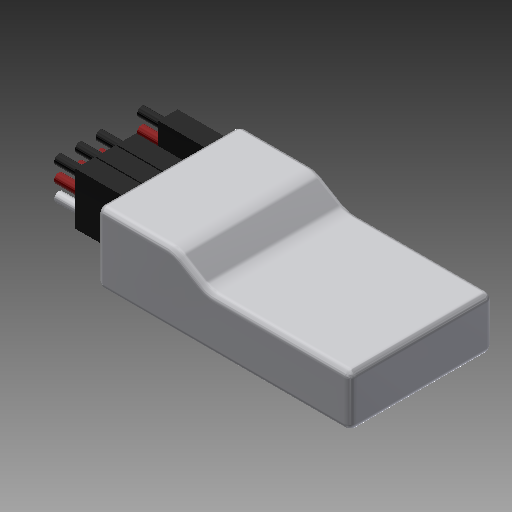
# Autodesk Inventor part: 受信機
Saved by Autodesk Inventor 2020 (Build 240168000, 168)
## iProperties
Created: 2013-08-05
Part Number: 受信機
Material: 一般
Document SubType Name: Modeling
Designer: Kentaro2
Mass: 5 g
Surface Area: 27.3811 cm^2
Volume: 7.76151 cm^3
Density: 0.644204 g/cm^3
Appearance: 既定
Author: Kentaro2
Autodesk Inventor part; units mm, degrees
ref_plane "YZ Plane" through (0, 0, 0) normal (1, 0, 0) x (0, 1, 0)
ref_plane "XZ Plane" through (0, 0, 0) normal (0, 1, 0) x (-1, 0, 0)
ref_plane "XY Plane" through (0, 0, 0) normal (0, 0, 1) x (1, 0, 0)
sketch "スケッチ1" plane through (0, 0, 0) normal (0, 0, 1) x (1, 0, 0)
  line L0 (-19.5, 11) -> (-19.5, 0)
  line L1 (-19.5, 0) -> (19.5, 0)
  line L2 (19.5, 0) -> (19.5, 8)
  line L3 (19.5, 8) -> (-2.5, 8)
  line L4 (-2.5, 8) -> (-7.5, 11)
  line L5 (-7.5, 11) -> (-19.5, 11)
  point P0 (0, 0)
  point P1 (0, 0)
  dimension "d0" = 8
  dimension "d1" = 11
  dimension "d2" = 39
  dimension "d3" = 12
  dimension "d4" = 22
  constraints: 12 end point, 3 parallel, 1 coincident, 1 horizontal, 1 midpoint, 1 perpendicular
  measures "d0" distance between parallel lines of L1 L3
  measures "d1" distance between parallel lines of L1 L5
  measures "d2" distance between parallel lines of L2 L0
  measures "d3" distance of L4.end L0.start
  measures "d4" distance of L2.end L3.end
extrude "押し出し1" add sketch "スケッチ1" along normal blind 22
fillet "フィレット1" radius 1 16 edges at (0, 0, 22) (8.5, 8, 22) (19.5, 4, 22) (-19.5, 0, 11) (0, 0, 0) (19.5, 0, 11) (19.5, 4, 0) (19.5, 8, 11) (-5, 9.5, 22) (8.5, 8, 0) (-5, 9.5, 0) (-13.5, 11, 22) (-19.5, 5.5, 22) (-13.5, 11, 0) (-19.5, 5.5, 0) (-19.5, 11, 11)
fillet "フィレット1" radius 4 2 edges at (-7.5, 11, 11) (-2.5, 8, 11)
sketch "スケッチ2" plane through (-19.5, 1, 1) normal (-1, 0, 0) x (0, 0, 1)
  line L0 (0, 0) -> (0, 9) projected
  line L1 (20, 0) -> (0, 0) projected
  line L2 (20, 9) -> (20, 0) projected
  line L3 (0.5347, 8.5347) -> (0.5347, 0.5347)
  line L4 (0.5347, 0.5347) -> (19.4653, 0.5347)
  line L5 (19.4653, 0.5347) -> (19.4653, 8.5)
  line L6 (0.5347, 8.5347) -> (3.5347, 8.5347)
  line L7 (3.5347, 8.5347) -> (3.5347, 0.5347)
  line L8 (3.5347, 0.5347) -> (0.5347, 0.5347)
  line L9 (0.5347, 0.5347) -> (0.5347, 8.5347)
  line L10 (3.7208, 8.5347) -> (6.7208, 8.5347)
  line L11 (6.7208, 8.5347) -> (6.7208, 0.5347)
  line L12 (6.7208, 0.5347) -> (3.7208, 0.5347)
  line L13 (3.7208, 0.5347) -> (3.7208, 8.5347)
  line L14 (6.9069, 8.5347) -> (9.9069, 8.5347)
  line L15 (9.9069, 8.5347) -> (9.9069, 0.5347)
  line L16 (9.9069, 0.5347) -> (6.9069, 0.5347)
  line L17 (6.9069, 0.5347) -> (6.9069, 8.5347)
  line L18 (10.0931, 8.5347) -> (13.0931, 8.5347)
  line L19 (13.0931, 8.5347) -> (13.0931, 0.5347)
  line L20 (13.0931, 0.5347) -> (10.0931, 0.5347)
  line L21 (10.0931, 0.5347) -> (10.0931, 8.5347)
  line L22 (13.2792, 8.5347) -> (16.2792, 8.5347)
  line L23 (16.2792, 8.5347) -> (16.2792, 0.5347)
  line L24 (16.2792, 0.5347) -> (13.2792, 0.5347)
  line L25 (13.2792, 0.5347) -> (13.2792, 8.5347)
  line L26 (16.4653, 8.5347) -> (19.4653, 8.5347)
  line L27 (19.4653, 8.5347) -> (19.4653, 0.5347)
  line L28 (19.4653, 0.5347) -> (16.4653, 0.5347)
  line L29 (16.4653, 0.5347) -> (16.4653, 8.5347)
  line L30 (3.5347, 8.5347) -> (3.7208, 8.5347)
  line L31 (6.7208, 8.5347) -> (6.9069, 8.5347)
  line L32 (9.9069, 8.5347) -> (10.0931, 8.5347)
  line L33 (13.0931, 8.5347) -> (13.2792, 8.5347)
  line L34 (16.2792, 8.5347) -> (16.4653, 8.5347)
  point P0 (-1, -1)
  dimension "d9" = 8
  dimension "d11" = 0.5347
  dimension "d12" = 3
  constraints: 64 end point, 16 equal length, 9 collinear, 7 perpendicular, 6 horizontal, 5 point on line, 2 other
  measures "d9" distance of L3.start L3.end
  measures "d11" distance between parallel lines of L0 L3
  measures "d12" distance between parallel lines of L7 L3
extrude "押し出し2" add sketch "スケッチ2" along normal blind 8 contours L6 L7 L4 L3 | L10 L11 L4 L13 | L14 L15 L4 L17 | L18 L19 L4 L21 | L22 L23 L4 L25 | L26 L27 L5 L4 L29
sketch "スケッチ4" plane through (-27.5, 1, 1) normal (-1, 0, 0) x (0, 0, 1)
  line L0 (0.5347, 8.5347) -> (0.5347, 0.5347) projected
  line L1 (6.7208, 0.5347) -> (6.7208, 8.5347) projected
  line L2 (6.7208, 8.5347) -> (3.7208, 8.5347) projected
  line L3 (3.7208, 8.5347) -> (3.7208, 0.5347) projected
  line L4 (3.7208, 0.5347) -> (6.7208, 0.5347) projected
  line L5 (9.9069, 0.5347) -> (9.9069, 8.5347) projected
  line L6 (9.9069, 8.5347) -> (6.9069, 8.5347) projected
  line L7 (6.9069, 8.5347) -> (6.9069, 0.5347) projected
  line L8 (6.9069, 0.5347) -> (9.9069, 0.5347) projected
  line L9 (13.0931, 0.5347) -> (13.0931, 8.5347) projected
  line L10 (13.0931, 8.5347) -> (10.0931, 8.5347) projected
  line L11 (10.0931, 8.5347) -> (10.0931, 0.5347) projected
  line L12 (10.0931, 0.5347) -> (13.0931, 0.5347) projected
  line L13 (16.2792, 0.5347) -> (16.2792, 8.5347) projected
  line L14 (16.2792, 8.5347) -> (13.2792, 8.5347) projected
  line L15 (13.2792, 8.5347) -> (13.2792, 0.5347) projected
  line L16 (13.2792, 0.5347) -> (16.2792, 0.5347) projected
  line L17 (19.4653, 0.5347) -> (19.4653, 8.5347) projected
  line L18 (19.4653, 8.5347) -> (16.4653, 8.5347) projected
  line L19 (16.4653, 8.5347) -> (16.4653, 0.5347) projected
  line L20 (16.4653, 0.5347) -> (19.4653, 0.5347) projected
  line L21 (1.0347, 3.5347) -> (1.0347, 5.5347)
  line L22 (1.0347, 1.0347) -> (1.0347, 3.0347)
  line L23 (1.0347, 7.3573) -> (0.5347, 7.3573)
  line L24 (1.3567, 6.0347) -> (1.3567, 5.5347)
  line L25 (1.3567, 3.5347) -> (1.3567, 3.0347)
  circle A0 centre (2.0347, 2.0347) radius 0.75
  circle A1 centre (2.0347, 4.5347) radius 0.75
  circle A2 centre (2.0347, 7.0347) radius 0.75
  circle A3 centre (5.2208, 7.0347) radius 0.75
  circle A4 centre (5.2208, 4.5347) radius 0.75
  circle A5 centre (5.2208, 2.0347) radius 0.75
  circle A6 centre (8.4069, 7.0347) radius 0.75
  circle A7 centre (8.4069, 4.5347) radius 0.75
  circle A8 centre (8.4069, 2.0347) radius 0.75
  circle A9 centre (11.5931, 2.0347) radius 0.75
  circle A10 centre (11.5931, 4.5347) radius 0.75
  circle A11 centre (11.5931, 7.0347) radius 0.75
  circle A12 centre (14.7792, 7.0347) radius 0.75
  circle A13 centre (14.7792, 4.5347) radius 0.75
  circle A14 centre (14.7792, 2.0347) radius 0.75
  circle A15 centre (17.9653, 2.0347) radius 0.75
  circle A16 centre (17.9653, 4.5347) radius 0.75
  circle A17 centre (17.9653, 7.0347) radius 0.75
  point P0 (-1, -1)
  dimension "d17" = 1.5
  constraints: 18 centre point, 17 equal radius, 10 end point, 2 collinear, 2 equal length, 1 coincident, 1 perpendicular, 1 point on line, 2 other
  measures "d17" diameter of A0
extrude "押し出し3" add sketch "スケッチ4" along normal blind 4 contours A0 | A1 | A2 | A3 | A4 | A5 | A6 | A7 | A8 | A9 | A10 | A11 | A12 | A13 | A14 | A15 | A16 | A17
sketch "スケッチ5" plane through (-31.5, 3.0347, 6.2208) normal (-1, 0, 0) x (0, 0, 1)
  line L0 (14.2445, 6.5) -> (14.2445, -1.5) projected
  circle A0 centre (12.7445, 2.5) radius 0.75 projected
  circle A1 centre (12.7445, 0) radius 0.75 projected
  circle A2 centre (12.7445, 5) radius 0.75 projected
  line L1 (14.2445, -1.5) -> (14.2445, 6.5) projected
  line L2 (14.2445, 6.5) -> (11.2445, 6.5) projected
  line L3 (11.2445, 6.5) -> (11.2445, -1.5) projected
  line L4 (11.2445, -1.5) -> (14.2445, -1.5) projected
  circle A3 centre (0, 2.5) radius 0.75 projected
  circle A4 centre (0, 5) radius 0.75 projected
  circle A5 centre (0, 0) radius 0.75 projected
  line L5 (1.5, -1.5) -> (1.5, 6.5) projected
  line L6 (1.5, 6.5) -> (-1.5, 6.5) projected
  line L7 (-1.5, 6.5) -> (-1.5, -1.5) projected
  line L8 (-1.5, -1.5) -> (1.5, -1.5) projected
  point P0 (-6.2208, -3.0347)
extrude "押し出し4" cut sketch "スケッチ5" against normal blind 12 contours L0 L4 L3 L2 | A0 | A1 | A2 | A3 | A4 | A5 | L8 L7 L6 L5
